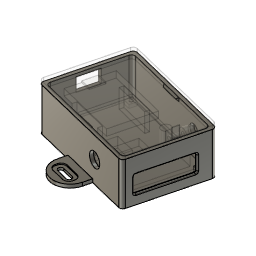
Enclosure v5 (Autodesk Fusion 360 design; units mm, degrees)
Autodesk Fusion 360 part; units mm, degrees
sketch "Sketch1" plane through (0, 0, 0) normal (0, 0, 1) x (1, 0, 0) in component "Case"
  line L0 (0, 0) -> (40.3, 0)
  line L1 (40.3, 0) -> (40.3, 60.25)
  line L2 (40.3, 60.25) -> (0, 60.25)
  line L3 (0, 60.25) -> (0, 0)
  line L4 (-3, 63.25) -> (-3, -3)
  line L5 (-3, -3) -> (43.3, -3)
  line L6 (43.3, -3) -> (43.3, 63.25)
  line L7 (43.3, 63.25) -> (-3, 63.25)
  circle A0 centre (38.55, 58.25) radius 0.9
  circle A1 centre (1.75, 58.25) radius 0.9
  line L8 (0, 60.25) -> (4, 60.25)
  line L9 (4, 60.25) -> (4, 56.25)
  line L10 (4, 56.25) -> (0, 56.25)
  line L11 (0, 56.25) -> (0, 60.25)
  line L12 (20.15, -3) -> (20.15, 63.25) construction
  line L13 (43.3, 30.125) -> (-3, 30.125) construction
  line L14 (36.3, 60.25) -> (36.3, 56.25)
  line L15 (36.3, 56.25) -> (40.3, 56.25)
  line L16 (4, 4) -> (0, 4)
  line L17 (4, 0) -> (4, 4)
  line L18 (36.3, 0) -> (36.3, 4)
  line L19 (36.3, 4) -> (40.3, 4)
  line L20 (-1, -1) -> (41.3, -1)
  line L21 (41.3, -1) -> (41.3, 61.25)
  line L22 (41.3, 61.25) -> (-1, 61.25)
  line L23 (-1, 61.25) -> (-1, -1)
  line L24 (43.3, 40.125) -> (58.3, 40.125)
  line L25 (58.3, 40.125) -> (58.3, 20.125)
  line L26 (58.3, 20.125) -> (43.3, 20.125)
  line L27 (43.3, 20.125) -> (43.3, 40.125)
  line L28 (-3, 40.125) -> (-18, 40.125)
  line L29 (-18, 40.125) -> (-18, 20.125)
  line L30 (-18, 20.125) -> (-3, 20.125)
  line L31 (52.3, 35.125) -> (49.3, 35.125)
  line L32 (49.3, 35.125) -> (49.3, 25.125)
  line L33 (49.3, 25.125) -> (52.3, 25.125)
  line L34 (52.3, 25.125) -> (52.3, 35.125)
  line L35 (52.3, 35.125) -> (49.3, 25.125) construction
  line L36 (49.3, 35.125) -> (52.3, 25.125) construction
  line L37 (-12, 35.125) -> (-9, 35.125)
  line L38 (-12, 25.125) -> (-12, 35.125)
  line L39 (-9, 25.125) -> (-12, 25.125)
  line L40 (-9, 35.125) -> (-9, 25.125)
  line L41 (47.3, 23.125) -> (54.3, 23.125)
  line L42 (54.3, 23.125) -> (54.3, 37.125)
  line L43 (54.3, 37.125) -> (47.3, 37.125)
  line L44 (47.3, 37.125) -> (47.3, 23.125)
  line L45 (-14, 37.125) -> (-7, 37.125)
  line L46 (-7, 37.125) -> (-7, 23.125)
  line L47 (-14, 23.125) -> (-14, 37.125)
  line L48 (-7, 23.125) -> (-14, 23.125)
  point P0 (43.3, 30.125)
  point P1 (50.8, 30.125)
  point P2 (-10.5, 30.125)
  point P3 (50.8, 30.125)
  dimension "d5" = 40.3
  dimension "d6" = 60.25
  dimension "d7" = 3
  dimension "d9" = 1.8
  dimension "d10" = 2
  dimension "d11" = 1.75
  dimension "d12" = 1.8
  dimension "d13" = 2
  dimension "d14" = 1.75
  dimension "d15" = 4
  dimension "d16" = 4
  dimension "d35" = 1
  dimension "d153" = 15
  dimension "d154" = 20
  dimension "d158" = 7.5
  dimension "d159" = 10
  dimension "d160" = 3
  dimension "d161" = 10
  dimension "d164" = 2
  constraint horizontal L0
  constraint vertical L1
  constraint horizontal L2
  constraint vertical L3
  constraint coincident L0.start L3.end
  constraint horizontal L8
  constraint vertical L9
  constraint horizontal L10
  constraint vertical L11
  constraint midpoint L5 L12.start
  constraint midpoint L7 L12.end
  constraint midpoint L6 P0
  constraint midpoint L4 L13.end
  constraint symmetric L8.end L12 L14.start
  constraint symmetric L9.end L12 L14.end
  constraint symmetric L10.end L12 L15.end
  constraint symmetric L8.end L13 L17.start
  constraint symmetric L9.end L13 L16.start
  constraint symmetric L10.end L13 L16.end
  constraint symmetric L13 L14.start L18.start
  constraint symmetric L13 L14.end L18.end
  constraint symmetric L13 L15.end L19.end
  constraint horizontal L24
  constraint vertical L25
  constraint horizontal L26
  constraint vertical L27
  constraint midpoint L27 P0
  constraint coincident P0 L13.start
  constraint symmetric L12 L24.start L28.start
  constraint symmetric L12 L24.end L28.end
  constraint symmetric L12 L25.end L29.end
  constraint symmetric L12 L26.end L30.end
  constraint symmetric L12 P3 P2
  constraint horizontal L31
  constraint perpendicular L31 L32
  constraint parallel L31 L33
  constraint parallel L32 L34
  constraint coincident L35 P3
  constraint coincident L36 P3
  constraint coincident P3 P1
  constraint symmetric L12 L31.start L37.start
  constraint symmetric L12 L31.end L37.end
  constraint symmetric L12 L32.end L39.start
  constraint symmetric L12 L33.end L38.start
  constraint symmetric L12 L41.start L46.end
  constraint symmetric L12 L41.end L47.start
  constraint symmetric L12 L42.end L45.start
  constraint symmetric L12 L43.end L45.end
  measures "d5" distance of L0.start L0.end
  measures "d6" distance of L0.start L2.end
  measures "d9" diameter of A0
  measures "d10" distance of L2 A0.centre
  measures "d11" distance of L1 A0.centre
  measures "d12" diameter of A1
  measures "d13" distance of L2 A1.centre
  measures "d14" distance of L3 A1.centre
  measures "d15" distance of L2.end L8.end
  measures "d16" distance of L2.end L10.end
  measures "d153" distance of L24.start L24.end
  measures "d154" distance of L24.start L26.end
  measures "d158" distance of L27 P3
  measures "d159" distance of L26 P3
  measures "d160" distance of L32.end L33.end
  measures "d161" distance of L31.end L32.end
extrude "Extrude1" add sketch "Sketch1" against normal blind 2 contours L0 L3 L16 L17 | L0 L1 L2 L3 L9 L10 L14 L15 L16 L17 L18 L19 | L0 L1 L18 L19 | L2 L3 L8 L9 L10 L11 | L1 L2 L14 L15 | L4 L5 L6 L7 L27 | L4 L28 L29 L30 | L6 L24 L25 L26 L27 | A0 | A1 | L20 L21 L22 L23 | L41 L42 L43 L44 | L45 L46 L47 L48 makes body 1 in component "Case"
extrude "Extrude2" add sketch "Sketch1" along normal blind 23 contours L4 L5 L6 L7 L27 bodies 1 in component "Case"
extrude "Extrude3" add sketch "Sketch1" along normal blind 2 contours L0 L3 L16 L17 | L0 L1 L18 L19 | L2 L3 L8 L9 L10 L11 | L1 L2 L14 L15 bodies 1 in component "Case"
sketch "Sketch1 (2)" plane through (0, 0, 23) normal (0, 0, 1) x (-1, 0, 0) in component "Lid"
  line L0 (-43.3, -63.25) -> (3, -63.25)
  line L1 (-43.3, -63.25) -> (3, -63.25)
  line L2 (3, -63.25) -> (3, 3)
  line L3 (3, 3) -> (-43.3, 3)
  line L4 (-43.3, 3) -> (-43.3, -63.25)
  line L5 (1, -61.25) -> (-41.3, -61.25)
  line L6 (-41.3, -61.25) -> (-41.3, 1)
  line L7 (-41.3, 1) -> (1, 1)
  line L8 (1, 1) -> (1, -61.25)
extrude "Extrude3'" add sketch "Sketch1 (2)" along normal blind 2 separate body contours L0 L1 L2 L3 L4 | L5 L6 L7 L8 makes body 2 in component "Lid"
extrude "Extrude4" add sketch "Sketch1 (2)" against normal blind 2 contours L5 L6 L7 L8 bodies 2 in component "Lid"
fillet "Fillet3" radius 2 4 edges at (-1, 61.25, 11.5) (41.3, 61.25, 11.5) (41.3, -1, 11.5) (-1, -1, 11.5) on bodies 1 in component "Case"
fillet "Fillet3'" radius 2 4 edges at (-1, 61.25, 22) (41.3, 61.25, 22) (41.3, -1, 22) (-1, -1, 22) on bodies 2 in component "Lid"
sketch "Sketch PerfBoard" plane through (0, 0, 0) normal (0, 0, 1) x (1, 0, 0) in component "PerfBoardPart"
  line L0 (0, 0) -> (40.3, 0)
  line L1 (40.3, 0) -> (40.3, 60.25)
  line L2 (40.3, 60.25) -> (0, 60.25)
  line L3 (0, 60.25) -> (0, 0)
  line L4 (20.15, 60.25) -> (20.15, 0) construction
  line L5 (40.3, 30.125) -> (0, 30.125) construction
  circle A0 centre (1.75, 58.25) radius 1
  circle A1 centre (38.55, 58.25) radius 1
  circle A2 centre (1.75, 2) radius 1
  circle A3 centre (38.55, 2) radius 1
  dimension "d36" = 40.3
  dimension "d37" = 60.25
  dimension "d39" = 2
  dimension "d40" = 2
  dimension "d41" = 1.75
  constraint horizontal L0
  constraint vertical L1
  constraint horizontal L2
  constraint vertical L3
  constraint coincident L0.start L3.end
  constraint midpoint L2 L4.start
  constraint midpoint L0 L4.end
  constraint midpoint L1 L5.start
  constraint midpoint L3 L5.end
  constraint symmetric L4 A0 A1
  constraint symmetric L5 A0 A2
  constraint symmetric L5 A1 A3
  measures "d36" distance of L0.start L0.end
  measures "d37" distance of L0.start L2.end
  measures "d39" diameter of A0
  measures "d40" distance of L2 A0.centre
  measures "d41" distance of L3 A0.centre
extrude "Extrude1'" add sketch "Sketch PerfBoard" along normal blind 1.6 separate body makes body 3 in component "PerfBoardPart"
sketch "Sketch Components" plane through (0, 0, 1.6) normal (0, 0, 1) x (-1, 0, 0) in component "PerfBoardPart"
  circle A0 centre (-1.75, -58.25) radius 1
  circle A1 centre (-1.75, -2) radius 1
  circle A2 centre (-38.55, -58.25) radius 1
  circle A3 centre (-38.55, -2) radius 1
  line L0 (0, -60.25) -> (0, 0)
  line L1 (0, 0) -> (-40.3, 0)
  line L2 (-40.3, 0) -> (-40.3, -60.25)
  line L3 (-40.3, -60.25) -> (0, -60.25)
  line L4 (-7, -53.5) -> (-9.37, -53.5)
  line L5 (-9.37, -53.5) -> (-9.37, -32.86)
  line L6 (-9.37, -32.86) -> (-7, -32.86)
  line L7 (-7, -32.86) -> (-7, -53.5)
  line L8 (-29.85, -53.5) -> (-32.22, -53.5)
  line L9 (-32.22, -53.5) -> (-32.22, -32.86)
  line L10 (-32.22, -32.86) -> (-29.85, -32.86)
  line L11 (-29.85, -32.86) -> (-29.85, -53.5)
  line L12 (-3.34, -2.59) -> (-33.84, -2.59)
  line L13 (-33.84, -2.59) -> (-33.84, -10.39)
  line L14 (-33.84, -10.39) -> (-3.34, -10.39)
  line L15 (-3.34, -10.39) -> (-3.34, -2.59)
  line L16 (-1, -26.15) -> (-23.14, -26.15)
  line L17 (-23.14, -26.15) -> (-23.14, -11)
  line L18 (-23.14, -11) -> (-1, -11)
  line L19 (-1, -11) -> (-1, -26.15)
  line L20 (-1, -18.575) -> (-23.14, -18.575) construction
  line L21 (-12.93, -15.475) -> (1.2, -15.475)
  line L22 (1.2, -15.475) -> (1.2, -21.675)
  line L23 (1.2, -21.675) -> (-12.93, -21.675)
  line L24 (-12.93, -21.675) -> (-12.93, -15.475)
  line L25 (-12.93, -15.475) -> (1.2, -21.675) construction
  line L26 (1.2, -15.475) -> (-12.93, -21.675) construction
  line L27 (-11.865, -24.575) -> (0.135, -24.575)
  line L28 (0.135, -24.575) -> (0.135, -12.575)
  line L29 (0.135, -12.575) -> (-11.865, -12.575)
  line L30 (-11.865, -12.575) -> (-11.865, -24.575)
  line L31 (-11.865, -24.575) -> (0.135, -12.575) construction
  line L32 (0.135, -24.575) -> (-11.865, -12.575) construction
  line L33 (-40.3, -15) -> (-29.3, -15)
  line L34 (-29.3, -15) -> (-29.3, -9)
  line L35 (-29.3, -9) -> (-40.3, -9)
  line L36 (-40.3, -9) -> (-40.3, -15)
  circle A4 centre (-30.65, -16.85) radius 2.65
  point P0 (-5.865, -18.575)
  point P1 (-5.865, -18.575)
  point P2 (-40.3, -12)
  dimension "d44" = 2.37
  dimension "d45" = 20.64
  dimension "d46" = 7
  dimension "d47" = 6.75
  dimension "d48" = 2.37
  dimension "d49" = 20.64
  dimension "d50" = 20.48
  dimension "d51" = 30.5
  dimension "d52" = 7.8
  dimension "d53" = 3.34
  dimension "d54" = 2.59
  dimension "d95" = 22.14
  dimension "d96" = 15.15
  dimension "d97" = 11
  dimension "d98" = 1
  dimension "d99" = 14.13
  dimension "d100" = 6.2
  dimension "d101" = 2.2
  dimension "d111" = 12
  dimension "d112" = 12
  dimension "d114" = 11
  dimension "d115" = 6
  dimension "d116" = 12
  dimension "d137" = 5.3
  dimension "d139" = 7
  dimension "d140" = 14.2
  constraint horizontal L4
  constraint vertical L5
  constraint horizontal L6
  constraint vertical L7
  constraint horizontal L8
  constraint vertical L9
  constraint horizontal L10
  constraint vertical L11
  constraint collinear L4 L8
  constraint horizontal L12
  constraint vertical L13
  constraint horizontal L14
  constraint vertical L15
  constraint horizontal L16
  constraint vertical L17
  constraint horizontal L18
  constraint vertical L19
  constraint midpoint L19 L20.start
  constraint midpoint L17 L20.end
  constraint horizontal L21
  constraint perpendicular L21 L22
  constraint parallel L21 L23
  constraint parallel L22 L24
  constraint coincident L25 P1
  constraint coincident L26 P1
  constraint coincident L20 P1
  constraint horizontal L27
  constraint perpendicular L27 L28
  constraint parallel L27 L29
  constraint parallel L28 L30
  constraint coincident L31 P1
  constraint coincident L32 P1
  constraint coincident P1 P0
  constraint horizontal L33
  constraint vertical L34
  constraint horizontal L35
  constraint vertical L36
  constraint midpoint L36 P2
  constraint coincident L2 L33.start
  measures "d44" distance of L4.start L4.end
  measures "d45" distance of L4.start L6.end
  measures "d46" distance of L0 L7
  measures "d47" distance of L3 L4
  measures "d48" distance of L8.start L8.end
  measures "d49" distance of L8.start L10.end
  measures "d50" distance of L5 L11
  measures "d51" distance of L12.start L12.end
  measures "d52" distance of L12.start L14.end
  measures "d53" distance of L0 L15
  measures "d54" distance of L1 L12
  measures "d95" distance of L16.start L16.end
  measures "d96" distance of L16.start L18.end
  measures "d97" distance of L1 L18
  measures "d98" distance of L0 L19
  measures "d99" distance of L22.end L23.end
  measures "d100" distance of L21.end L22.end
  measures "d101" distance of L19 L22
  measures "d111" distance of L28.end L29.end
  measures "d112" distance of L27.end L28.end
  measures "d114" distance of L33.start L33.end
  measures "d115" distance of L33.start L35.end
  measures "d116" distance of L1 P2
  measures "d137" diameter of A4
  measures "d139" distance of L2 A4
  measures "d140" distance of L1 A4
extrude "Extrude2'" add sketch "Sketch Components" along normal blind 9.74 contours L13 L14 L34 L35 | L12 L13 L14 L15 L34 L35 bodies 3 in component "PerfBoardPart"
extrude "Extrude3''" add sketch "Sketch Components" along normal blind 11.08 contours L4 L5 L6 L7 | L8 L9 L10 L11 bodies 3 in component "PerfBoardPart"
sketch "Sketch Wemos" plane through (0, 0, 12.68) normal (0, 0, 1) x (-1, 0, 0) in component "PerfBoardPart"
  line L0 (-7, -32.86) -> (-9.37, -32.86)
  line L1 (-9.37, -32.86) -> (-9.37, -53.5)
  line L2 (-9.37, -53.5) -> (-7, -53.5)
  line L3 (-7, -53.5) -> (-7, -32.86)
  line L4 (-7, -59.98) -> (-32.32, -59.98)
  line L5 (-32.32, -59.98) -> (-32.32, -25.65)
  line L6 (-32.32, -25.65) -> (-7, -25.65)
  line L7 (-7, -25.65) -> (-7, -59.98)
  line L8 (-7, -32.86) -> (-7, -53.5)
  line L9 (-7, -53.5) -> (-9.37, -53.5)
  line L10 (-19.66, -59.98) -> (-19.66, -25.65) construction
  line L11 (-15.56, -59.98) -> (-23.76, -59.98)
  line L12 (-23.76, -59.98) -> (-23.76, -53.98)
  line L13 (-23.76, -53.98) -> (-15.56, -53.98)
  line L14 (-15.56, -53.98) -> (-15.56, -59.98)
  point P0 (-19.66, -59.98)
  dimension "d59" = 25.32
  dimension "d60" = 34.33
  dimension "d61" = 6.48
  dimension "d143" = 8.2
  dimension "d144" = 6
  constraint horizontal L4
  constraint vertical L5
  constraint horizontal L6
  constraint vertical L7
  constraint collinear L7 L8
  constraint midpoint L4 P0
  constraint midpoint L6 L10.end
  constraint horizontal L11
  constraint vertical L12
  constraint horizontal L13
  constraint vertical L14
  constraint midpoint L11 P0
  constraint coincident P0 L10.start
  measures "d59" distance of L4.start L4.end
  measures "d60" distance of L4.start L6.end
  measures "d61" distance of L4 L9
  measures "d143" distance of L11.start L11.end
  measures "d144" distance of L11.start L13.end
extrude "Extrude Wemos" add sketch "Sketch Wemos" along normal blind 3.74 bodies 3 in component "PerfBoardPart"
extrude "Extrude4'" cut 1 faces at (13.5067, 2.59, 4.8467) faces seen with x (1, 0, 0) y (0, 1, 0) z (0, 0, 1) at (0, 0, 2) along direction (0, -1, 0) up to surface (5.59 mm away) on bodies 3 bodies 1 in component "Case"
fillet "Fillet4" radius 2 4 edges at (-3, -3, 10.5) (43.3, -3, 10.5) (43.3, 63.25, 10.5) (-3, 63.25, 10.5) on bodies 1 in component "Case"
fillet "Fillet4'" radius 2 4 edges at (-3, -3, 24) (43.3, -3, 24) (43.3, 63.25, 24) (-3, 63.25, 24) on bodies 2 in component "Lid"
fillet "Fillet5" radius 0.8 2 faces at (13.5067, -1.6667, 13.34) (13.5067, -1.6667, 3.6) on bodies 1 in component "Case"
fillet "Fillet5" radius 0.8 2 faces at (3.34, -1.6667, 6.8467) (33.84, -1.6667, 6.8467) on bodies 1 in component "Case"
sketch "Sketch3" plane through (41.3, 0, 0) normal (-1, 0, 0) x (0, -1, 0) in component "Case"
  line L0 (-1, 0) -> (-1, 23)
  line L1 (-1, 23) -> (-59.25, 23)
  line L2 (-59.25, 23) -> (-59.25, 0)
  line L3 (-59.25, 0) -> (-1, 0)
  line L4 (-36.125, 23) -> (-24.125, 23)
  line L5 (-24.125, 23) -> (-24.125, 21)
  line L6 (-24.125, 21) -> (-36.125, 21)
  line L7 (-36.125, 21) -> (-36.125, 23)
  line L8 (-30.125, 23) -> (-30.125, 21) construction
  line L9 (-30.125, 23) -> (-30.125, 21) construction
  dimension "d80" = 12
  dimension "d81" = 2
  dimension "d86" = 2
  constraint horizontal L4
  constraint vertical L5
  constraint horizontal L6
  constraint vertical L7
  constraint coincident L1 L4.start
  constraint midpoint L1 L8.start
  constraint perpendicular L1 L8
  constraint midpoint L4 L8.start
  constraint midpoint L6 L8.end
  constraint collinear L8 L9
  measures "d80" distance of L4.start L4.end
  measures "d81" distance of L4.start L6.end
  measures "d86" distance of L8.start L8.end
extrude "Extrude Clasp Void" cut sketch "Sketch3" along normal blind 2.6 draft -45 contours L1 L4 L5 L6 L7 bodies 2 in component "Lid"
extrude "Extrude5" add sketch "Sketch3" along normal blind 2 draft -45 contours L1 L4 L5 L6 L7 bodies 1 in component "Case"
ref_plane "WorkPlane1" through (20.15, 30.125, 11.5) normal (-1, 0, 0) x (0, -1, 0) in component "Case"
mirror "Mirror1" about plane through (20.15, 30.125, 11.5) normal (-1, 0, 0) of "Extrude5" in component "Case"
extrude "Extrude5'" add sketch "Sketch Components" along normal blind 4 contours L19 L23 L27 L30 | L16 L17 L18 L19 L21 L23 L24 L27 L29 L30 | L19 L21 L23 L30 | L19 L21 L29 L30 | L21 L23 L24 L30 bodies 3 in component "PerfBoardPart"
extrude "Extrude6" add sketch "Sketch Components" along normal blind 6 from surface at 4 contours L0 L19 L21 L23 | L0 L21 L23 L28 | L19 L23 L27 L30 | L21 L22 L23 L28 | L19 L21 L23 L30 | L19 L21 L29 L30 bodies 3 in component "PerfBoardPart"
sketch "Sketch 3.5mm Port" plane through (-1.2, 0, 0) normal (-1, 0, 0) x (0, -1, 0) in component "PerfBoardPart"
  line L0 (-21.675, 5.6) -> (-15.475, 5.6)
  line L1 (-15.475, 5.6) -> (-15.475, 11.6)
  line L2 (-15.475, 11.6) -> (-21.675, 11.6)
  line L3 (-21.675, 11.6) -> (-21.675, 5.6)
  circle A0 centre (-18.575, 8.6) radius 3
  dimension "d107" = 6
  measures "d107" diameter of A0
extrude "Extrude7" cut sketch "Sketch 3.5mm Port" against normal up to surface (2.2 mm away) contours L0 L2 L3 A0 | L0 L1 L2 A0 bodies 3 in component "PerfBoardPart"
extrude "Extrude Antenna Port" add sketch "Sketch Components" along normal blind 6 from surface at 7 contours L2 L13 L14 L33 L34 L35 L36 A4 bodies 3 in component "PerfBoardPart"
sketch "Sketch5" plane through (40.3, 0, 0) normal (1, 0, 0) x (0, 1, 0) in component "PerfBoardPart"
  line L0 (9, 8.6) -> (15, 8.6)
  line L1 (15, 8.6) -> (15, 14.6)
  line L2 (15, 14.6) -> (9, 14.6)
  line L3 (9, 14.6) -> (9, 8.6)
  circle A0 centre (12, 11.6) radius 3
  dimension "d120" = 6
  measures "d120" diameter of A0
extrude "Extrude9" cut sketch "Sketch5" against normal blind 4.3 contours L0 L3 A0 | L0 L1 A0 | L2 L3 A0 | L1 L2 A0 bodies 3 in component "PerfBoardPart"
sketch "Sketch6" plane through (29.3, 0, 0) normal (-1, 0, 0) x (0, -1, 0) in component "PerfBoardPart"
  line L0 (-10.39, 14.6) -> (-14.5696, 14.6)
  line L1 (-14.5696, 8.6) -> (-10.39, 8.6)
  line L2 (-10.39, 8.6) -> (-10.39, 11.34)
  circle A0 centre (-12, 11.6) radius 1.25
  line L3 (-10.39, 11.34) -> (-10.39, 14.6)
  line L4 (-14.5696, 14.6) -> (-14.5696, 8.6)
  dimension "d123" = 2.5
  measures "d123" diameter of A0
extrude "Extrude10" cut sketch "Sketch6" against normal up to surface (6.7 mm away) bodies 3 in component "PerfBoardPart"
extrude "Extrude11" cut 1 faces at (35.28, 9.4633, 14.6) along direction (0, 0, -1) up to surface (6 mm away) on bodies 3 bodies 3 makes body 4 at (26.1167, 39.2113, 0) in component "PerfBoardPart"
extrude "Extrude6'" cut 1 faces at (-1.2, 18.8114, 7.9002) faces seen with x (1, 0, 0) y (0, 1, 0) z (0, 0, 1) at (0, 0, 2) along direction (-1, 0, 0) up to surface (1.8 mm away) and the other way blind 1 on bodies 4 bodies 1 in component "Case"
move_face "OffsetFaces1" offset -1.15 1 faces at (-2.3333, 18.7245, 13.5963) on bodies 1 in component "Case"
extrude "Extrude7'" cut 1 faces at (40.3, 12.6235, 11.0215) faces seen with x (1, 0, 0) y (0, 1, 0) z (0, 0, 1) at (0, 0, 2) along direction (1, 0, 0) up to surface (3 mm away) on bodies 3 bodies 1 in component "Case"
extrude "Extrude12" add sketch "Sketch Components" along normal blind 12.2 contours L33 L34 A4 picked at (-31.3029, -17.6075) bodies 4 in component "PerfBoardPart"
extrude "Extrude13" add sketch "Sketch Wemos" along normal blind 3.6 from surface at 1 contours L4 L11 L12 L13 L14 bodies 4 in component "PerfBoardPart"
sketch "Sketch MicroUSB Port" plane through (0, 59.98, 0) normal (0, 1, 0) x (-1, 0, 0) in component "PerfBoardPart"
  line L0 (-32.32, 12.68) -> (-7, 12.68)
  line L1 (-7, 12.68) -> (-7, 16.42)
  line L2 (-7, 16.42) -> (-15.56, 16.42)
  line L3 (-15.56, 16.42) -> (-15.56, 17.28)
  line L4 (-15.56, 17.28) -> (-23.76, 17.28)
  line L5 (-23.76, 17.28) -> (-23.76, 16.42)
  line L6 (-23.76, 16.42) -> (-32.32, 16.42)
  line L7 (-32.32, 16.42) -> (-32.32, 12.68)
  line L8 (-23.76, 17.28) -> (-15.56, 17.28)
  line L9 (-23.76, 16.42) -> (-23.76, 17.28)
  line L10 (-15.56, 16.42) -> (-15.56, 17.28)
  line L11 (-23.76, 17.28) -> (-15.56, 17.28)
  line L12 (-15.56, 17.28) -> (-15.56, 13.28)
  line L13 (-15.56, 13.28) -> (-23.76, 13.28)
  line L14 (-23.76, 13.28) -> (-23.76, 17.28)
  dimension "d148" = 4
  constraint horizontal L11
  constraint vertical L12
  constraint horizontal L13
  constraint vertical L14
  constraint coincident L4.end L5.start
  measures "d148" distance of L4.end L13.end
extrude "Extrude8" cut sketch "Sketch MicroUSB Port" along normal up to surface (3.27 mm away) contours L3 L4 L5 L8 L9 L10 L11 L12 L13 L14 sketch seen with x (1, 0, 0) y (0, 1, 0) z (0, 0, 1) at (0, 0, 2) bodies 1 in component "Case"
move_face "OffsetFaces2" offset -2 4 faces at (23.76, 61.9167, 17.9467) (18.2933, 61.9167, 15.28) (15.56, 61.9167, 17.9467) (18.2933, 61.9167, 19.28) on bodies 1 in component "Case"
move_face "OffsetFaces3" offset -0.2 1 faces at (41.9667, 14.9851, 13.8987) on bodies 1 in component "Case"
extrude "Extrude9'" cut sketch "Sketch1" against normal blind 0.6667 contours L41 L42 L43 L44 | L45 L46 L47 L48 bodies 1 in component "Case"
fillet "Fillet7" radius 10 4 edges at (58.3, 20.125, -1) (58.3, 40.125, -1) (-18, 20.125, -1) (-18, 40.125, -1) on bodies 1 in component "Case"
fillet "Fillet7" radius 1.5 8 edges at (-12, 35.125, -1.3333) (-9, 35.125, -1.3333) (-9, 25.125, -1.3333) (-12, 25.125, -1.3333) (49.3, 35.125, -1.3333) (49.3, 25.125, -1.3333) (52.3, 25.125, -1.3333) (52.3, 35.125, -1.3333) on bodies 1 in component "Case"
fillet "Fillet7" radius 3 8 edges at (47.3, 37.125, -0.3333) (54.3, 37.125, -0.3333) (54.3, 23.125, -0.3333) (47.3, 23.125, -0.3333) (-14, 37.125, -0.3333) (-7, 37.125, -0.3333) (-7, 23.125, -0.3333) (-14, 23.125, -0.3333) on bodies 1 in component "Case"
ref_plane "WorkPlane1" through (20.15, 47.6875, 22) normal (1, 0, 0) x (0, -1, 0) in component "Lid"
mirror "Mirror1'" [suppressed] in component "Lid"
move_face "OffsetFaces1'" [suppressed] in component "Lid"
shell "Shell1" [suppressed] in component "Lid"
delete_face "DeleteFace1" [suppressed] in component "Lid"
delete_face "DeleteFace2" [suppressed] in component "Lid"
component "Case" placed x (1, 0, 0) y (0, 1, 0) z (0, 0, 1) at (0, 0, 0)
component "Lid" placed x (1, 0, 0) y (0, 1, 0) z (0, 0, 1) at (0, 0, 0)
component "PerfBoardPart" placed x (1, 0, 0) y (0, 1, 0) z (0, 0, 1) at (0, 0, 2)
equation "board_width = 40.3 mm"
equation "board_length = 60.25 mm"
equation "enclosure_height = 23 mm"
equation "wall_thickness = 2 mm"
equation "d5 = board_width"
equation "d6 = board_length"
equation "d7 = wall_thickness + 1 mm"
equation "mount_hold_diam = 1.8 mm"
equation "d9 = mount_hold_diam"
equation "d12 = mount_hold_diam"
equation "d17 = -wall_thickness"
equation "d19 = enclosure_height"
equation "d21 = wall_thickness"
equation "d36 = board_width"
equation "d37 = board_length"
equation "d66 = wall_thickness"
equation "d68 = -wall_thickness"
equation "d92 = wall_thickness"
equation "d153 = mount_ear_dimension"
equation "mount_ear_dimension = 15 mm"
equation "d158 = mount_ear_dimension / 2"
equation "d159 = d154 / 2"
equation "d160 = screwslot_width"
equation "d163 = screwslot_width / 2"
equation "screwslot_width = 3 mm"
equation "d166 = -wall_thickness * ( 1 / 3 )"
equation "d169 = screwslot_width"
named bodies: "Case", "Project_Envelope", "Lid", "Project_Envelope (1)"
